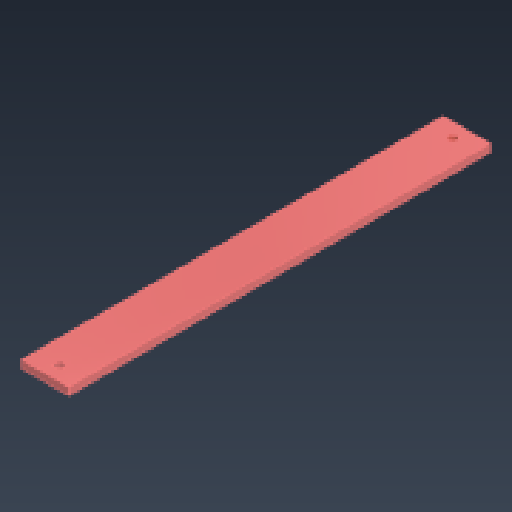
# Autodesk Inventor part: жгут низ
Saved by Autodesk Inventor 2026 (Build 300175000, 175)
## iProperties
Created: 2026-01-20
Part Number: жгут низ
Material: Типовые
Document SubType Name: Modeling
Designer: GameHD
Density: 1 g/cm^3
Appearance: Гладкий — красный
Author: GameHD
Autodesk Inventor part; units mm, degrees
ref_plane "YZ Plane" through (0, 0, 0) normal (1, 0, 0) x (0, 1, 0)
ref_plane "XZ Plane" through (0, 0, 0) normal (0, 1, 0) x (-1, 0, 0)
ref_plane "XY Plane" through (0, 0, 0) normal (0, 0, 1) x (1, 0, 0)
sketch "Эскиз1" plane through (0, 0, 0) normal (0, 1, 0) x (-1, 0, 0)
  line L0 (0, 0) -> (25, 0)
  line L1 (25, 0) -> (25, 222)
  line L2 (25, 222) -> (0, 222)
  line L3 (0, 222) -> (0, 0)
  dimension "d0" = 25
  dimension "d1" = 222
  constraints: 8 end point, 2 parallel, 1 horizontal, 1 perpendicular
  measures "d0" distance of L2.end L1.end
  measures "d1" distance of L1.end L0.end
extrude "Выдавливание1" add sketch "Эскиз1" along normal blind 4
sketch "Эскиз2" plane through (0, 4, 0) normal (0, 1, 0) x (1, 0, 0)
  circle A0 centre (-12.5, -7.5) radius 2.25
  line L0 (0, 0) -> (-25, 0) projected
  line L1 (0, -222) -> (0, 0) projected
  line L2 (0, -111) -> (-46.0375, -111)
  circle A1 centre (-12.5, -214.5) radius 2.25
  dimension "d4" = 4.5
  dimension "d5" = 7.5
  constraints: 2 centre point, 2 end point, 1 horizontal, 1 midpoint, 1 symmetric about line, 1 other
  measures "d4" diameter of A0
  measures "d5" distance from line of L0 A0.centre
extrude "Выдавливание2" cut sketch "Эскиз2" against normal blind 4
